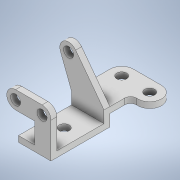
# Autodesk Inventor part: Pieza4Miniproyecto
Saved by Autodesk Inventor 2021 (Build 250183000, 183)
## iProperties
Created: 2021-02-26
Part Number: Pieza4Miniproyecto
Material: Genérico
Document SubType Name: Modeling
Designer: Arturo
Density: 1 g/cm^3
Appearance: Valor por defecto
Author: Arturo
Autodesk Inventor part; units mm, degrees
ref_plane "YZ Plane" through (0, 0, 0) normal (1, 0, 0) x (0, 1, 0)
ref_plane "XZ Plane" through (0, 0, 0) normal (0, 1, 0) x (-1, 0, 0)
ref_plane "XY Plane" through (0, 0, 0) normal (0, 0, 1) x (1, 0, 0)
sketch "Boceto1" plane through (0, 0, 0) normal (0, 1, 0) x (-1, 0, 0)
  line L0 (0, 0) -> (110, 0)
  line L1 (110, 0) -> (110, -200)
  line L2 (110, -200) -> (0, -200)
  line L3 (0, -200) -> (0, 0)
  circle A0 centre (55, -100) radius 17
  dimension "d0" = 110
  dimension "d1" = 200
  constraints: 8 end point, 2 parallel, 1 centre point, 1 horizontal, 1 perpendicular
  measures "d0" distance of L1.end L2.end
  measures "d1" distance of L0.end L1.end
extrude "Extrusión1" add sketch "Boceto1" along normal blind 20
sketch "Boceto2" plane through (-110, 0, 0) normal (0, 0, 1) x (1, 0, 0)
  line L0 (110, 20) -> (0, 20) projected
  line L1 (0, 20) -> (55, 20)
  line L2 (110, 0) -> (0, 0) projected
  line L3 (110, 20) -> (110, 120)
  circle A0 centre (80, 120) radius 17
  arc A1 (110, 120) -> (80, 150) centre (80, 120) ccw
  circle A2 centre (-10, 120) radius 17
  arc A3 (-10, 150) -> (-10, 90) centre (-10, 120) ccw
  line L4 (-10, 90) -> (55, 90)
  line L5 (55, 90) -> (55, 20)
  line L6 (-10, 150) -> (80, 150)
  dimension "d8" = 55
  constraints: 10 end point, 4 centre point, 4 point on circle, 2 coincident, 2 perpendicular, 2 tangent, 1 horizontal, 1 midpoint, 1 vertical
  measures "d8" distance of L0.end L1.end
extrude "Extrusión2" add sketch "Boceto2" against normal blind 20
sketch "Boceto3" plane through (0, 0, -200) normal (0, 0, -1) x (-1, 0, 0)
  line L0 (110, 20) -> (0, 20)
  line L1 (0, 20) -> (0, 60)
  line L2 (0, 60) -> (110, 60)
  line L3 (110, 60) -> (110, 20)
  point P0 (0, 0)
  dimension "d19" = 110
  dimension "d20" = 40
  constraints: 8 end point, 2 parallel, 1 horizontal, 1 perpendicular
  measures "d19" distance of L1.end L2.end
  measures "d20" distance of L0.end L1.end
extrude "Extrusión3" add sketch "Boceto3" against normal blind 20
sketch "Boceto4" plane through (0, 0, -200) normal (0, 0, -1) x (-1, 0, 0)
  line L0 (0, 0) -> (110, 0) projected
  line L1 (110, 0) -> (110, 60) projected
  circle A0 centre (120, 170) radius 17
  arc A1 (148.016, 159.2713) -> (96, 188) centre (120, 170) ccw
  line L2 (110, 60) -> (148.016, 159.2713)
  line L3 (0, 60) -> (96, 188)
  line L4 (0, 60) -> (110, 60) projected
  line L5 (0, 60) -> (110, 60)
  constraints: 6 end point, 2 centre point, 2 point on circle, 2 tangent, 1 coincident, 1 collinear
extrude "Extrusión4" add sketch "Boceto4" against normal blind 20
sketch "Boceto5" plane through (0, 0, 0) normal (1, 0, 0) x (0, 0, -1)
  line L0 (0, 0) -> (200, 0) projected
  line L1 (200, 0) -> (200, 60) projected
  line L2 (200, 60) -> (180, 60) projected
  line L3 (180, 20) -> (180, 60) projected
  line L4 (20, 20) -> (180, 20) projected
  line L5 (20, 120) -> (20, 20) projected
  line L6 (0, 120) -> (20, 120) projected
  line L7 (0, 0) -> (0, 120) projected
  line L8 (180, 20) -> (180, 60) projected
  line L9 (180, 60) -> (310, 60)
  line L10 (310, 60) -> (310, 40)
  line L11 (310, 40) -> (180, 40)
  line L12 (180, 40) -> (180, 60)
  dimension "d30" = 130
  dimension "d31" = 20
  constraints: 8 end point, 2 parallel, 1 horizontal, 1 perpendicular
  measures "d30" distance of L10.end L11.end
  measures "d31" distance of L9.end L10.end
extrude "Extrusión5" add sketch "Boceto5" against normal blind 110 contours L11 L3 L2 L1 | L1 L9 L10 L11
sketch "Boceto6" plane through (0, 60, -200) normal (0, 1, 0) x (1, 0, 0)
  line L0 (0, 0) -> (-110, 0) projected
  line L1 (0, 110) -> (0, 0) projected
  line L2 (0, 110) -> (-110, 110) projected
  line L3 (-110, 0) -> (-110, 110) projected
  line L4 (-96, 0) -> (0, 0) projected
  line L5 (0, 0) -> (0, 110) projected
  line L6 (0, 0) -> (0, 50.2087)
  line L7 (0, 110) -> (-70, 110)
  line L8 (0, 110) -> (-110, 110) projected
  circle A0 centre (-70, 110) radius 17
  arc A1 (-70, 150) -> (-110, 110) centre (-70, 110) ccw
  arc A2 (21.6667, 70.1391) -> (25, 150) centre (25, 110) ccw
  circle A3 centre (25, 110) radius 17
  line L9 (25, 150) -> (-70, 150)
  arc A4 (21.6667, 70.1391) -> (0, 50.2087) centre (20, 50.2087) ccw
  line L10 (-110, 110) -> (-110, 0) projected
  line L11 (-110, 110) -> (-110, 50.2087)
  line L12 (-110, 50.2087) -> (0, 50.2087)
  point P0 (0, -200)
  point P1 (0, 78.775)
  point P2 (-110, 50.2087)
  point P3 (-87, 110)
  point P4 (-53, 110)
  dimension "d41" = 20
  constraints: 10 end point, 7 point on circle, 5 centre point, 5 point on line, 4 tangent, 3 coincident, 1 collinear, 1 perpendicular
  measures "d41" radius of A4
extrude "Extrusión6" add sketch "Boceto6" against normal blind 20 contours L12 L3 L2 A0 L1 | L1 L2 A0 A1 L9 A2 A4
extrude "Extrusión7" cut sketch "Boceto6" against normal blind 20 contours A0 L2 picked at (-58.8313, 108.6439)
